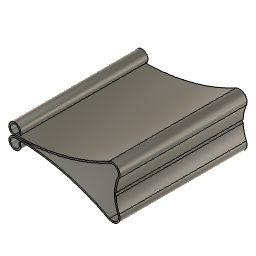
Binder Clip (Autodesk Fusion 360 design; units mm, degrees)
Autodesk Fusion 360 part; units mm, degrees
sketch "Sketch1" plane through (0, 0, 0) normal (0, 1, 0) x (1, 0, 0)
  line L0 (0, 0) -> (27.4351, 0) construction
  line L1 (27.4351, 0) -> (27.4351, -6.156) construction
  line L2 (27.4351, -6.156) -> (0, -6.156) construction
  line L3 (0, -6.156) -> (0, 0) construction
  arc A0 (25.2234, -5.9764) -> (1.5, 0.01) centre (1.5, -49.99) ccw
  arc A1 (26.4351, 0) -> (27.3028, -4.04) centre (36.2741, 0) ccw
  line L4 (26.4351, 0) -> (26.4351, -4) construction
  line L5 (26.4351, 0) -> (27.4351, 0) construction
  line L6 (1.5, 0.01) -> (1.5, 0) construction
  line L7 (1.5, -1.49) -> (1.5, -0.99) construction
  line L8 (1.5, -0.99) -> (2.8098, -0.759) construction
  arc A2 (1.6729, 0) -> (2.8098, -0.759) centre (1.5, -1.49) ccw
  arc A3 (2.8098, -0.759) -> (1.6729, 0) centre (1.5, -1.49) ccw construction
  arc A4 (26.4351, -3.2417) -> (25.2234, -5.9764) centre (25.9351, -4.656) ccw construction
  arc A5 (25.2234, -5.9764) -> (27.4351, -4.656) centre (25.9351, -4.656) ccw
  arc A6 (27.3028, -4.04) -> (26.4351, -3.2417) centre (25.9351, -4.656) ccw construction
  arc A7 (27.4351, -4.656) -> (27.3028, -4.04) centre (25.9351, -4.656) ccw
  line L9 (26.8124, -0.37) -> (27.4351, -0.37) construction
  arc A8 (26.8124, -0.37) -> (27.6402, -3.8881) centre (36.2741, 0) ccw
  arc A9 (27.8051, -4.656) -> (27.6402, -3.8881) centre (25.9351, -4.656) ccw
  arc A10 (25.0479, -6.3021) -> (27.8051, -4.656) centre (25.9351, -4.656) ccw
  arc A11 (25.0479, -6.3021) -> (1.5, -0.36) centre (1.5, -49.99) ccw
  arc A12 (1.6303, -0.3675) -> (2.4868, -0.9393) centre (1.5, -1.49) ccw
  line L10 (2.4868, -0.9393) -> (2.8098, -0.759)
  line L11 (1.5542, -0.36) -> (1.4494, -0.3611)
  line L12 (1.5542, -0.36) -> (1.4494, -0.3611)
  line L13 (26.8124, -0.37) -> (26.4351, 0)
  arc A13 (1.5, -0.01) -> (25.2234, 5.9764) centre (1.5, 49.99) ccw
  arc A14 (27.4351, 4.656) -> (25.2234, 5.9764) centre (25.9351, 4.656) ccw
  arc A15 (27.3028, 4.04) -> (27.4351, 4.656) centre (25.9351, 4.656) ccw
  arc A16 (27.3028, 4.04) -> (26.4351, 0) centre (36.2741, 0) ccw
  line L14 (26.8124, 0.37) -> (26.4351, 0)
  arc A17 (27.6402, 3.8881) -> (26.8124, 0.37) centre (36.2741, 0) ccw
  arc A18 (27.6402, 3.8881) -> (27.8051, 4.656) centre (25.9351, 4.656) ccw
  arc A19 (27.8051, 4.656) -> (25.0479, 6.3021) centre (25.9351, 4.656) ccw
  arc A20 (1.5, 0.36) -> (25.0479, 6.3021) centre (1.5, 49.99) ccw
  line L15 (2.4868, 0.9393) -> (2.8098, 0.759)
  arc A21 (2.4868, 0.9393) -> (1.6303, 0.3675) centre (1.5, 1.49) ccw
  arc A22 (2.8098, 0.759) -> (1.6729, 0) centre (1.5, 1.49) ccw
  dimension "d6" = 3
  dimension "d7" = 3
  dimension "d8" = 50
  dimension "d9" = 4
  dimension "d10" = 1
  dimension "d11" = 0.01
  dimension "d12" = 0.5
  dimension "d13" = 100
  dimension "d14" = -0.37
  dimension "d15" = -0.37
  constraint horizontal L0
  constraint vertical L1
  constraint horizontal L2
  constraint vertical L3
  constraint coincident L0.start L3.end
  constraint tangent L2 A5
  constraint tangent L1 A5
  constraint tangent L3 A2
  constraint coincident A0.end A2
  constraint tangent A0 A5
  constraint tangent A0 A2
  constraint coincident L0 A1.start
  constraint coincident A1.end A5
  constraint tangent A1 A5
  constraint perpendicular L0 L4
  constraint tangent A1 L4
  constraint vertical L7.start A0.end
  constraint coincident L0 L6.end
  constraint perpendicular L0 L6
  constraint coincident L7.start A2.centre
  constraint vertical L7
  constraint coincident L0 A2.start
  constraint concentric A2 A3
  constraint coincident L4 A4.start
  constraint concentric A4 A5
  constraint coincident L1 A5.end
  constraint concentric A5 A6
  constraint concentric A5 A7
  constraint coincident A11 L11.start
  constraint coincident A12 L11.end
  constraint parallel L11 L12
  constraint tangent A11 A12
  constraint symmetric L0 A0.end A13.start
  constraint symmetric L0 A0.start A13.end
  constraint symmetric L0 A0 A13
  constraint symmetric L0 A1.end A15.start
  constraint symmetric L0 A1.start L4.start
  constraint symmetric L0 A1 A16
  constraint symmetric L0 L8.end L15.end
  constraint symmetric L0 A2.start A3.end
  constraint symmetric L0 A2 A22
  constraint symmetric L0 A5.end A14.start
  constraint symmetric L0 A5 A14
  constraint symmetric L0 A7 A15
  constraint symmetric L0 L9.start L14.start
  constraint symmetric L0 A8.end A17.start
  constraint symmetric L0 A8 A17
  constraint symmetric L0 A9.start A18.end
  constraint symmetric L0 A9 A18
  constraint symmetric L0 A10.start A19.end
  constraint symmetric L0 A10 A19
  constraint symmetric L0 A11.end A20.start
  constraint symmetric L0 A11 A20
  constraint symmetric L0 A12.start A21.end
  constraint symmetric L0 A12.end L15.start
  constraint symmetric L0 A12 A21
  measures "d6" diameter of A5
  measures "d7" diameter of A2
  measures "d8" radius of A0
  measures "d9" distance of A1.start L4.end
  measures "d10" distance of L0.end A1.start
  measures "d11" distance of A0.end L6.end
  measures "d12" distance of L7.start L7.end
  measures "d13" angle of L7 L8
extrude "Extrude1" add sketch "Sketch1" along normal mid plane 31.8 contours A0 A1 A2 A5 A7 A8 A9 A10 A11 A12 L10 L11 L12 L13 A13 A22 | A0 A2 A13 A14 A15 A16 L14 A17 A18 A19 A20 L15 A21 A22
equation "height = 18.9 mm"
equation "length = 31.9 mm"
equation "clip_height = 37.0 mm"
equation "clip_width = 15.9 mm"
equation "bottom_width = 6.5 mm"
equation "d16 = clip_width"
